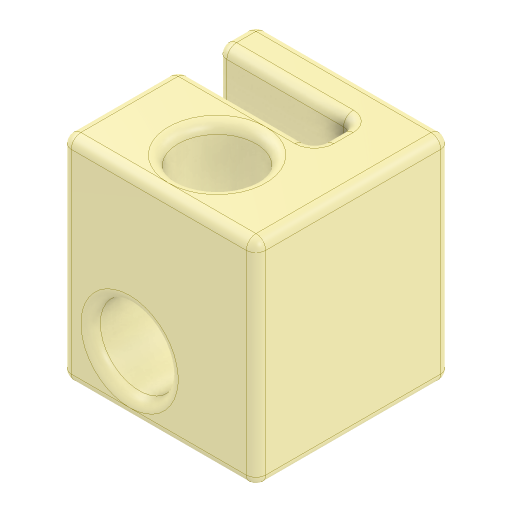
# Autodesk Inventor part: ProbeSharpener
Saved by Autodesk Inventor 2023 (Build 270158000, 158)
## iProperties
Created: 2022-01-24
Part Number: ProbeSharpener
Material: Generic
Document SubType Name: Modeling
Designer: Pip
Density: 1 g/cm^3
Appearance: Nylon 6
Author: Pip
Autodesk Inventor part; units mm, degrees
ref_plane "YZ Plane" through (0, 0, 0) normal (1, 0, 0) x (0, 1, 0)
ref_plane "XZ Plane" through (0, 0, 0) normal (0, 1, 0) x (-1, 0, 0)
ref_plane "XY Plane" through (0, 0, 0) normal (0, 0, 1) x (1, 0, 0)
sketch "Sketch1" plane through (0, 0, 0) normal (0, 1, 0) x (-1, 0, 0)
  line L0 (5, -5) -> (-5, -5)
  line L1 (-5, -5) -> (-5, 5)
  line L2 (-5, 5) -> (5, 5)
  line L3 (5, 5) -> (5, -5)
  point P0 (0, 0)
  dimension "d0" = 10
  dimension "d1" = 10
  dimension "d2" = 5
  dimension "d3" = 5
  constraints: 8 end point, 2 parallel, 1 horizontal, 1 perpendicular
  measures "d0" distance of L0.start L0.end
  measures "d1" distance of L2.end L0.start
  measures "d2" distance from line of point (0, 0) L2
  measures "d3" distance from line of point (0, 0) L1
extrude "Extrusion1" add sketch "Sketch1" along normal blind 10
sketch "Sketch2" plane through (0, 10, 0) normal (0, 1, 0) x (1, 0, 0)
  line L0 (5, -5) -> (5, 5) projected
  line L1 (-5, -5) -> (5, -5) projected
  point P0 (0, -2)
  point P1 (0, -2)
  dimension "d30" = 5
  dimension "d31" = 3
  constraints: 1 coincident
  measures "d30" distance from line of L0 point (0, -2)
  measures "d31" distance from line of L1 point (0, -2)
hole "Hole1" at (0, 10, 2) direction (0, -1, 0) diameter 4 depth 4.8 tip angle 118
sketch "Sketch3" plane through (0, 0, 0) normal (0, -1, 0) x (1, 0, 0)
  line L0 (5, -5) -> (-5, -5) projected
  line L1 (5, 5) -> (5, -5) projected
  line L2 (-5, -5) -> (5, -5)
  line L3 (5, -5) -> (5, -3)
  line L4 (5, -3) -> (-5, -3)
  line L5 (-5, -3) -> (-5, -5)
  line L6 (5, -3) -> (2, -3)
  line L7 (2, -3) -> (2, -1)
  line L8 (2, -1) -> (5, -1)
  line L9 (5, -1) -> (5, -3)
  line L10 (-5, -5) -> (-5, 5) projected
  line L11 (5, -1) -> (-5, -1)
  line L12 (-5, -1) -> (-5, 5)
  line L13 (-5, 5) -> (5, 5)
  line L14 (5, 5) -> (5, -1)
  point P0 (0, 0)
  dimension "d13" = 2
  dimension "d14" = 3
  dimension "d15" = 2
  constraints: 24 end point, 6 parallel, 3 horizontal, 3 perpendicular, 1 point on line
  measures "d13" distance of L3.end L2.end
  measures "d14" distance of L7.end L8.end
  measures "d15" distance of L6.end L7.end
extrude "Extrusion2" add sketch "Sketch3" along normal blind 1 contours L0 L5 L4 L1 | L4 L7 L8 L1 | L8 L11 L10 L13 L1
sketch "Sketch4" plane through (-5, 10, 5) normal (0, 0, 1) x (1, 0, 0)
  line L0 (0, -10) -> (7, -10) projected
  line L1 (0, -10) -> (0, -11) projected
  line L2 (7, -11) -> (0, -11) projected
  line L3 (7, -10) -> (7, -11) projected
  point P0 (5, -10)
  point P1 (3.5, -8)
  dimension "d18" = 7
  dimension "d19" = 3.5
  dimension "d20" = 3
  measures "d18" distance of L2.start L1.end
  measures "d19" distance from line of point (3.5, -8) L3
  measures "d20" distance from line of L2 point (3.5, -8)
hole "Hole2" at (-1.5, 2, 5) direction (0, 0, -1) diameter 4 depth 6 tip angle 118
sketch "Sketch5" plane through (0, 0, 0) normal (0, -1, 0) x (1, 0, 0)
  line L0 (2, -1) -> (-1.5, -1) projected
  line L1 (-5, -3) -> (-5, -1) projected
  line L2 (-5, -3) -> (2, -3) projected
  line L3 (2, -3) -> (2, -1) projected
  line L4 (-1.5, -1) -> (-5, -1) projected
  line L5 (2, -1) -> (0.2321, -1) projected
  line L6 (-5, -3) -> (2, -3)
  line L7 (2, -3) -> (2, -1)
  line L8 (2, -1) -> (-5, -1)
  line L9 (-5, -1) -> (-5, -3)
  point P0 (0, 0)
  constraints: 8 end point, 2 parallel, 1 horizontal, 1 perpendicular
extrude "Extrusion3" cut sketch "Sketch5" against normal through all
fillet "Fillet1" radius 0.5 3 edges at (2, 4.5, -3) (2, 4.5, -1) (0, 5.2, 0)
fillet "Fillet1" radius 0.5 25 edges at (-5, 10, -4) (-5, 4.5, -3) (-5, -1, -4) (-5, 4.5, -5) (-1.5, -1, -3) (-1.5, 10, -3) (0, 10, -5) (5, 10, 0) (0, 10, 5) (-5, 10, 2) (-1.5, 10, -1) (2, 10, -2) (0, 10, 0) (0, -1, -5) (5, 4.5, -5) (2, -1, -2) (-1.5, -1, -1) (-5, -1, 2) (0, -1, 5) (5, -1, 0) (5, 4.5, 5) (-5, 4.5, 5) (-1.5, 4, 5) (-5, 4.5, -1) (-1.5, 4, -1)
equation "\"d2\" = 0.5 * d1"
equation "\"d3\" = 0.5 * d0"
equation "\"d19\" = 0.5 * d18"
body "Solid1"
